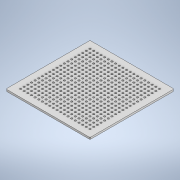
# Autodesk Inventor part: MouldCover20x20
Saved by Autodesk Inventor 2020.3 (Build 243373010, 373A)
## iProperties
Created: 2020-10-26
Part Number: MouldCover20x20
Material: Generic
Document SubType Name: Modeling
Designer: Naude Conradie
Density: 1 g/cm^3
Appearance: Default
Author: Naude Conradie
Autodesk Inventor part; units mm, degrees
ref_plane "YZ Plane" through (0, 0, 0) normal (1, 0, 0) x (0, 1, 0)
ref_plane "XZ Plane" through (0, 0, 0) normal (0, 1, 0) x (-1, 0, 0)
ref_plane "XY Plane" through (0, 0, 0) normal (0, 0, 1) x (1, 0, 0)
sketch "Sketch1" plane through (0, 0, 0) normal (0, 1, 0) x (-1, 0, 0)
  line L0 (0, 0) -> (230, 0)
  line L1 (230, 0) -> (230, -230)
  line L2 (230, -230) -> (0, -230)
  line L3 (0, -230) -> (0, 0)
  dimension "d0" = 230
  dimension "d1" = 230
  constraints: 8 end point, 2 parallel, 1 horizontal, 1 perpendicular
  measures "d0" distance of L1.end L2.end
  measures "d1" distance of L0.end L1.end
extrude "Extrusion1" add sketch "Sketch1" along normal blind 5
sketch "Sketch2" plane through (0, 5, 0) normal (0, 1, 0) x (1, 0, 0)
  line L0 (-230, 0) -> (0, 0) projected
  line L1 (0, 0) -> (0, 230) projected
  point P0 (-20, 20)
  point P1 (-30, 20)
  point P2 (-40, 20)
  point P3 (-50, 20)
  point P4 (-60, 20)
  point P5 (-70, 20)
  point P6 (-80, 20)
  point P7 (-90, 20)
  point P8 (-100, 20)
  point P9 (-110, 20)
  point P10 (-120, 20)
  point P11 (-130, 20)
  point P12 (-140, 20)
  point P13 (-150, 20)
  point P14 (-160, 20)
  point P15 (-170, 20)
  point P16 (-180, 20)
  point P17 (-190, 20)
  point P18 (-200, 20)
  point P19 (-210, 20)
  point P20 (-20, 30)
  point P21 (-30, 30)
  point P22 (-40, 30)
  point P23 (-50, 30)
  point P24 (-60, 30)
  point P25 (-70, 30)
  point P26 (-80, 30)
  point P27 (-90, 30)
  point P28 (-100, 30)
  point P29 (-110, 30)
  point P30 (-120, 30)
  point P31 (-130, 30)
  point P32 (-140, 30)
  point P33 (-150, 30)
  point P34 (-160, 30)
  point P35 (-170, 30)
  point P36 (-180, 30)
  point P37 (-190, 30)
  point P38 (-200, 30)
  point P39 (-210, 30)
  point P40 (-20, 40)
  point P41 (-30, 40)
  point P42 (-40, 40)
  point P43 (-50, 40)
  point P44 (-60, 40)
  point P45 (-70, 40)
  point P46 (-80, 40)
  point P47 (-90, 40)
  point P48 (-100, 40)
  point P49 (-110, 40)
  point P50 (-120, 40)
  point P51 (-130, 40)
  point P52 (-140, 40)
  point P53 (-150, 40)
  point P54 (-160, 40)
  point P55 (-170, 40)
  point P56 (-180, 40)
  point P57 (-190, 40)
  point P58 (-200, 40)
  point P59 (-210, 40)
  point P60 (-20, 50)
  point P61 (-30, 50)
  point P62 (-40, 50)
  point P63 (-50, 50)
  point P64 (-60, 50)
  point P65 (-70, 50)
  point P66 (-80, 50)
  point P67 (-90, 50)
  point P68 (-100, 50)
  point P69 (-110, 50)
  point P70 (-120, 50)
  point P71 (-130, 50)
  point P72 (-140, 50)
  point P73 (-150, 50)
  point P74 (-160, 50)
  point P75 (-170, 50)
  point P76 (-180, 50)
  point P77 (-190, 50)
  point P78 (-200, 50)
  point P79 (-210, 50)
  point P80 (-20, 60)
  point P81 (-30, 60)
  point P82 (-40, 60)
  point P83 (-50, 60)
  point P84 (-60, 60)
  point P85 (-70, 60)
  point P86 (-80, 60)
  point P87 (-90, 60)
  point P88 (-100, 60)
  point P89 (-110, 60)
  point P90 (-120, 60)
  point P91 (-130, 60)
  point P92 (-140, 60)
  point P93 (-150, 60)
  point P94 (-160, 60)
  point P95 (-170, 60)
  point P96 (-180, 60)
  point P97 (-190, 60)
  point P98 (-200, 60)
  point P99 (-210, 60)
  point P100 (-20, 70)
  point P101 (-30, 70)
  point P102 (-40, 70)
  point P103 (-50, 70)
  point P104 (-60, 70)
  point P105 (-70, 70)
  point P106 (-80, 70)
  point P107 (-90, 70)
  point P108 (-100, 70)
  point P109 (-110, 70)
  point P110 (-120, 70)
  point P111 (-130, 70)
  point P112 (-140, 70)
  point P113 (-150, 70)
  point P114 (-160, 70)
  point P115 (-170, 70)
  point P116 (-180, 70)
  point P117 (-190, 70)
  point P118 (-200, 70)
  point P119 (-210, 70)
  point P120 (-20, 80)
  point P121 (-30, 80)
  point P122 (-40, 80)
  point P123 (-50, 80)
  point P124 (-60, 80)
  point P125 (-70, 80)
  point P126 (-80, 80)
  point P127 (-90, 80)
  point P128 (-100, 80)
  point P129 (-110, 80)
  point P130 (-120, 80)
  point P131 (-130, 80)
  point P132 (-140, 80)
  point P133 (-150, 80)
  point P134 (-160, 80)
  point P135 (-170, 80)
  point P136 (-180, 80)
  point P137 (-190, 80)
  point P138 (-200, 80)
  point P139 (-210, 80)
  point P140 (-20, 90)
  point P141 (-30, 90)
  point P142 (-40, 90)
  point P143 (-50, 90)
  point P144 (-60, 90)
  point P145 (-70, 90)
  point P146 (-80, 90)
  point P147 (-90, 90)
  point P148 (-100, 90)
  point P149 (-110, 90)
  point P150 (-120, 90)
  point P151 (-130, 90)
  point P152 (-140, 90)
  point P153 (-150, 90)
  point P154 (-160, 90)
  point P155 (-170, 90)
  point P156 (-180, 90)
  point P157 (-190, 90)
  point P158 (-200, 90)
  point P159 (-210, 90)
  point P160 (-20, 100)
  point P161 (-30, 100)
  point P162 (-40, 100)
  point P163 (-50, 100)
  point P164 (-60, 100)
  point P165 (-70, 100)
  point P166 (-80, 100)
  point P167 (-90, 100)
  point P168 (-100, 100)
  point P169 (-110, 100)
  point P170 (-120, 100)
  point P171 (-130, 100)
  point P172 (-140, 100)
  point P173 (-150, 100)
  point P174 (-160, 100)
  point P175 (-170, 100)
  point P176 (-180, 100)
  point P177 (-190, 100)
  point P178 (-200, 100)
  point P179 (-210, 100)
  point P180 (-20, 110)
  point P181 (-30, 110)
  point P182 (-40, 110)
  point P183 (-50, 110)
  point P184 (-60, 110)
  point P185 (-70, 110)
  point P186 (-80, 110)
  point P187 (-90, 110)
  point P188 (-100, 110)
  point P189 (-110, 110)
  point P190 (-120, 110)
  point P191 (-130, 110)
  point P192 (-140, 110)
  point P193 (-150, 110)
  point P194 (-160, 110)
  point P195 (-170, 110)
  point P196 (-180, 110)
  point P197 (-190, 110)
  point P198 (-200, 110)
  point P199 (-210, 110)
  dimension "d4" = 20
  dimension "d5" = 20
  dimension "d8" = 10
  dimension "d11" = 10
  constraints: 1 horizontal, 1 vertical, 399 other
  measures "d4" distance from line of L0 point (-20, 20)
  measures "d5" distance from line of L1 point (-20, 20)
  measures "d8" distance of point (-20, 20) point (-30, 20)
  measures "d11" distance of point (-20, 20) point (-20, 30)
hole "Hole1" at (-20, 5, -20) at (-30, 5, -20) at (-40, 5, -20) at (-50, 5, -20) at (-60, 5, -20) at (-70, 5, -20) at (-80, 5, -20) at (-90, 5, -20) at (-100, 5, -20) at (-110, 5, -20) at (-120, 5, -20) at (-130, 5, -20) at (-140, 5, -20) at (-150, 5, -20) at (-160, 5, -20) at (-170, 5, -20) at (-180, 5, -20) at (-190, 5, -20) at (-200, 5, -20) at (-210, 5, -20) at (-20, 5, -30) at (-30, 5, -30) at (-40, 5, -30) at (-50, 5, -30) at (-60, 5, -30) at (-70, 5, -30) at (-80, 5, -30) at (-90, 5, -30) at (-100, 5, -30) at (-110, 5, -30) at (-120, 5, -30) at (-130, 5, -30) at (-140, 5, -30) at (-150, 5, -30) at (-160, 5, -30) at (-170, 5, -30) at (-180, 5, -30) at (-190, 5, -30) at (-200, 5, -30) at (-210, 5, -30) at (-20, 5, -40) at (-30, 5, -40) at (-40, 5, -40) at (-50, 5, -40) at (-60, 5, -40) at (-70, 5, -40) at (-80, 5, -40) at (-90, 5, -40) at (-100, 5, -40) at (-110, 5, -40) direction (0, -1, 0) diameter 5 end through all and at (-120, 5, -40) (-130, 5, -40) (-140, 5, -40) (-150, 5, -40) (-160, 5, -40) (-170, 5, -40) (-180, 5, -40) (-190, 5, -40) (-200, 5, -40) (-210, 5, -40) (-20, 5, -50) (-30, 5, -50) (-40, 5, -50) (-50, 5, -50) (-60, 5, -50) (-70, 5, -50) (-80, 5, -50) (-90, 5, -50) (-100, 5, -50) (-110, 5, -50) (-120, 5, -50) (-130, 5, -50) (-140, 5, -50) (-150, 5, -50) (-160, 5, -50) (-170, 5, -50) (-180, 5, -50) (-190, 5, -50) (-200, 5, -50) (-210, 5, -50) (-20, 5, -60) (-30, 5, -60) (-40, 5, -60) (-50, 5, -60) (-60, 5, -60) (-70, 5, -60) (-80, 5, -60) (-90, 5, -60) (-100, 5, -60) (-110, 5, -60) (-120, 5, -60) (-130, 5, -60) (-140, 5, -60) (-150, 5, -60) (-160, 5, -60) (-170, 5, -60) (-180, 5, -60) (-190, 5, -60) (-200, 5, -60) (-210, 5, -60) (-20, 5, -70) (-30, 5, -70) (-40, 5, -70) (-50, 5, -70) (-60, 5, -70) (-70, 5, -70) (-80, 5, -70) (-90, 5, -70) (-100, 5, -70) (-110, 5, -70) (-120, 5, -70) (-130, 5, -70) (-140, 5, -70) (-150, 5, -70) (-160, 5, -70) (-170, 5, -70) (-180, 5, -70) (-190, 5, -70) (-200, 5, -70) (-210, 5, -70) (-20, 5, -80) (-30, 5, -80) (-40, 5, -80) (-50, 5, -80) (-60, 5, -80) (-70, 5, -80) (-80, 5, -80) (-90, 5, -80) (-100, 5, -80) (-110, 5, -80) (-120, 5, -80) (-130, 5, -80) (-140, 5, -80) (-150, 5, -80) (-160, 5, -80) (-170, 5, -80) (-180, 5, -80) (-190, 5, -80) (-200, 5, -80) (-210, 5, -80) (-20, 5, -90) (-30, 5, -90) (-40, 5, -90) (-50, 5, -90) (-60, 5, -90) (-70, 5, -90) (-80, 5, -90) (-90, 5, -90) (-100, 5, -90) (-110, 5, -90) (-120, 5, -90) (-130, 5, -90) (-140, 5, -90) (-150, 5, -90) (-160, 5, -90) (-170, 5, -90) (-180, 5, -90) (-190, 5, -90) (-200, 5, -90) (-210, 5, -90) (-20, 5, -100) (-30, 5, -100) (-40, 5, -100) (-50, 5, -100) (-60, 5, -100) (-70, 5, -100) (-80, 5, -100) (-90, 5, -100) (-100, 5, -100) (-110, 5, -100) (-120, 5, -100) (-130, 5, -100) (-140, 5, -100) (-150, 5, -100) (-160, 5, -100) (-170, 5, -100) (-180, 5, -100) (-190, 5, -100) (-200, 5, -100) (-210, 5, -100) (-20, 5, -110) (-30, 5, -110) (-40, 5, -110) (-50, 5, -110) (-60, 5, -110) (-70, 5, -110) (-80, 5, -110) (-90, 5, -110) (-100, 5, -110) (-110, 5, -110) (-120, 5, -110) (-130, 5, -110) (-140, 5, -110) (-150, 5, -110) (-160, 5, -110) (-170, 5, -110) (-180, 5, -110) (-190, 5, -110) (-200, 5, -110) (-210, 5, -110) (-20, 5, -120) (-30, 5, -120) (-40, 5, -120) (-50, 5, -120) (-60, 5, -120) (-70, 5, -120) (-80, 5, -120) (-90, 5, -120) (-100, 5, -120) (-110, 5, -120) (-120, 5, -120) (-130, 5, -120) (-140, 5, -120) (-150, 5, -120) (-160, 5, -120) (-170, 5, -120) (-180, 5, -120) (-190, 5, -120) (-200, 5, -120) (-210, 5, -120) (-20, 5, -130) (-30, 5, -130) (-40, 5, -130) (-50, 5, -130) (-60, 5, -130) (-70, 5, -130) (-80, 5, -130) (-90, 5, -130) (-100, 5, -130) (-110, 5, -130) (-120, 5, -130) (-130, 5, -130) (-140, 5, -130) (-150, 5, -130) (-160, 5, -130) (-170, 5, -130) (-180, 5, -130) (-190, 5, -130) (-200, 5, -130) (-210, 5, -130) (-20, 5, -140) (-30, 5, -140) (-40, 5, -140) (-50, 5, -140) (-60, 5, -140) (-70, 5, -140) (-80, 5, -140) (-90, 5, -140) (-100, 5, -140) (-110, 5, -140) (-120, 5, -140) (-130, 5, -140) (-140, 5, -140) (-150, 5, -140) (-160, 5, -140) (-170, 5, -140) (-180, 5, -140) (-190, 5, -140) (-200, 5, -140) (-210, 5, -140) (-20, 5, -150) (-30, 5, -150) (-40, 5, -150) (-50, 5, -150) (-60, 5, -150) (-70, 5, -150) (-80, 5, -150) (-90, 5, -150) (-100, 5, -150) (-110, 5, -150) (-120, 5, -150) (-130, 5, -150) (-140, 5, -150) (-150, 5, -150) (-160, 5, -150) (-170, 5, -150) (-180, 5, -150) (-190, 5, -150) (-200, 5, -150) (-210, 5, -150) (-20, 5, -160) (-30, 5, -160) (-40, 5, -160) (-50, 5, -160) (-60, 5, -160) (-70, 5, -160) (-80, 5, -160) (-90, 5, -160) (-100, 5, -160) (-110, 5, -160) (-120, 5, -160) (-130, 5, -160) (-140, 5, -160) (-150, 5, -160) (-160, 5, -160) (-170, 5, -160) (-180, 5, -160) (-190, 5, -160) (-200, 5, -160) (-210, 5, -160) (-20, 5, -170) (-30, 5, -170) (-40, 5, -170) (-50, 5, -170) (-60, 5, -170) (-70, 5, -170) (-80, 5, -170) (-90, 5, -170) (-100, 5, -170) (-110, 5, -170) (-120, 5, -170) (-130, 5, -170) (-140, 5, -170) (-150, 5, -170) (-160, 5, -170) (-170, 5, -170) (-180, 5, -170) (-190, 5, -170) (-200, 5, -170) (-210, 5, -170) (-20, 5, -180) (-30, 5, -180) (-40, 5, -180) (-50, 5, -180) (-60, 5, -180) (-70, 5, -180) (-80, 5, -180) (-90, 5, -180) (-100, 5, -180) (-110, 5, -180) (-120, 5, -180) (-130, 5, -180) (-140, 5, -180) (-150, 5, -180) (-160, 5, -180) (-170, 5, -180) (-180, 5, -180) (-190, 5, -180) (-200, 5, -180) (-210, 5, -180) (-20, 5, -190) (-30, 5, -190) (-40, 5, -190) (-50, 5, -190) (-60, 5, -190) (-70, 5, -190) (-80, 5, -190) (-90, 5, -190) (-100, 5, -190) (-110, 5, -190) (-120, 5, -190) (-130, 5, -190) (-140, 5, -190) (-150, 5, -190) (-160, 5, -190) (-170, 5, -190) (-180, 5, -190) (-190, 5, -190) (-200, 5, -190) (-210, 5, -190) (-20, 5, -200) (-30, 5, -200) (-40, 5, -200) (-50, 5, -200) (-60, 5, -200) (-70, 5, -200) (-80, 5, -200) (-90, 5, -200) (-100, 5, -200) (-110, 5, -200) (-120, 5, -200) (-130, 5, -200) (-140, 5, -200) (-150, 5, -200) (-160, 5, -200) (-170, 5, -200) (-180, 5, -200) (-190, 5, -200) (-200, 5, -200) (-210, 5, -200) (-20, 5, -210) (-30, 5, -210) (-40, 5, -210) (-50, 5, -210) (-60, 5, -210) (-70, 5, -210) (-80, 5, -210) (-90, 5, -210) (-100, 5, -210) (-110, 5, -210) (-120, 5, -210) (-130, 5, -210) (-140, 5, -210) (-150, 5, -210) (-160, 5, -210) (-170, 5, -210) (-180, 5, -210) (-190, 5, -210) (-200, 5, -210) (-210, 5, -210)
chamfer "Chamfer1" distance 2 angle 45 4 edges at (-230, 2.5, -230) (0, 2.5, -230) (0, 2.5, 0) (-230, 2.5, 0)
body "Solid1"
